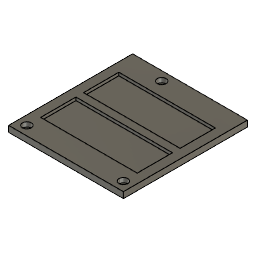
Final_Enclosure_Lid (Autodesk Fusion 360 design; units mm, degrees)
Autodesk Fusion 360 part; units mm, degrees
sketch "Sketch1" plane through (0, 0, 0) normal (0, 0, 1) x (1, 0, 0)
  line L0 (0, 0) -> (75, 0)
  line L1 (75, 0) -> (75, 81)
  line L2 (75, 81) -> (0, 81)
  line L3 (0, 81) -> (0, 0)
  dimension "d1" = 81
  dimension "d2" = 75
  constraint horizontal L0
  constraint vertical L1
  constraint horizontal L2
  constraint vertical L3
  constraint coincident L0.start L3.end
  measures "d1" distance of L0.start L2.end
  measures "d2" distance of L0.start L0.end
extrude "Extrude1" add sketch "Sketch1" along normal blind 4
sketch "Sketch2" plane through (0, 0, 0) normal (0, 0, -1) x (1, 0, 0)
  line L0 (0, 0) -> (0, -81)
  line L1 (0, -81) -> (75, -81)
  line L2 (75, -81) -> (75, 0)
  line L3 (75, 0) -> (0, 0)
  line L4 (72.95, -78.95) -> (2.05, -78.95)
  line L5 (2.05, -78.95) -> (2.05, -2.05)
  line L6 (2.05, -2.05) -> (72.95, -2.05)
  line L7 (72.95, -2.05) -> (72.95, -78.95)
  dimension "d6" = 2.05
  dimension "d7" = 2.05
  dimension "d8" = 2.05
  dimension "d9" = 2.05
  measures "d6" distance of L3 L6
  measures "d7" distance of L0 L5
  measures "d8" distance of L1 L4
  measures "d9" distance of L2 L7
extrude "Extrude2" add sketch "Sketch2" along normal blind 2 contours L4 L5 L6 L7
sketch "Sketch3" plane through (0, 0, 4) normal (0, 0, 1) x (-1, 0, 0)
  line L0 (0, -81) -> (0, 0)
  line L1 (0, 0) -> (-75, 0)
  line L2 (-75, 0) -> (-75, -81)
  line L3 (-75, -81) -> (0, -81)
  circle A0 centre (-6, -6) radius 2.875
  circle A1 centre (-69, -6) radius 2.875
  circle A2 centre (-25, -75) radius 2.875
  dimension "d12" = 25
  dimension "d13" = 5.75
  dimension "d14" = 6
  dimension "d15" = 6
  dimension "d16" = 6
  dimension "d17" = 6
  dimension "d18" = 6
  dimension "d19" = 5.75
  dimension "d20" = 5.75
  measures "d12" distance of L0 A2.centre
  measures "d13" diameter of A2
  measures "d14" distance of L3 A2.centre
  measures "d15" distance of L1 A0.centre
  measures "d16" distance of L1 A1.centre
  measures "d17" distance of L2 A1.centre
  measures "d18" distance of L0 A0.centre
  measures "d19" diameter of A0
  measures "d20" diameter of A1
extrude "Extrude3" cut sketch "Sketch3" against normal blind 3 contours A0 | A1 | A2
sketch "Sketch4" plane through (0, 0, 4) normal (0, 0, 1) x (-1, 0, 0)
  circle A0 centre (-25, -75) radius 2.875
  circle A1 centre (-6, -6) radius 2.875
  circle A2 centre (-69, -6) radius 2.875
  line L0 (0, -81) -> (0, 0)
  line L1 (0, 0) -> (-75, 0)
  line L2 (-75, 0) -> (-75, -81)
  line L3 (-75, -81) -> (0, -81)
  circle A3 centre (-6, -6) radius 1.55
  circle A4 centre (-69, -6) radius 1.55
  circle A5 centre (-25, -75) radius 1.55
  dimension "d23" = 3.1
  dimension "d24" = 3.1
  dimension "d25" = 3.1
  constraint concentric A1 A3
  constraint concentric A2 A4
  constraint concentric A0 A5
  measures "d23" diameter of A3
  measures "d24" diameter of A4
  measures "d25" diameter of A5
extrude "Extrude4" cut sketch "Sketch4" against normal blind 16 contours A3 | A4 | A5
sketch "Sketch5" plane through (0, 0, 4) normal (0, 0, 1) x (-1, 0, 0)
  circle A0 centre (-25, -75) radius 2.875
  circle A1 centre (-6, -6) radius 2.875
  circle A2 centre (-69, -6) radius 2.875
  line L0 (0, -81) -> (0, 0)
  line L1 (0, 0) -> (-75, 0)
  line L2 (-75, 0) -> (-75, -81)
  line L3 (-75, -81) -> (0, -81)
  line L4 (-69, -66) -> (-6, -66)
  line L5 (-6, -66) -> (-6, -43)
  line L6 (-6, -43) -> (-69, -43)
  line L7 (-69, -43) -> (-69, -66)
  line L8 (-69, -38) -> (-6, -38)
  line L9 (-6, -38) -> (-6, -15)
  line L10 (-6, -15) -> (-69, -15)
  line L11 (-69, -15) -> (-69, -38)
  dimension "d28" = 23
  dimension "d29" = 15
  dimension "d30" = 23
  dimension "d31" = 15
  dimension "d32" = 6
  dimension "d33" = 6
  dimension "d34" = 6
  dimension "d35" = 6
  constraint horizontal L4
  constraint vertical L5
  constraint horizontal L6
  constraint vertical L7
  constraint horizontal L8
  constraint vertical L9
  constraint horizontal L10
  constraint vertical L11
  measures "d28" distance of L4.start L6.end
  measures "d29" distance of L3 L4
  measures "d30" distance of L8.start L10.end
  measures "d31" distance of L1 L10
  measures "d32" distance of L2 L7
  measures "d33" distance of L2 L11
  measures "d34" distance of L0 L9
  measures "d35" distance of L0 L5
extrude "Extrude5" cut sketch "Sketch5" against normal blind 2 contours L4 L5 L6 L7 | L8 L9 L10 L11
